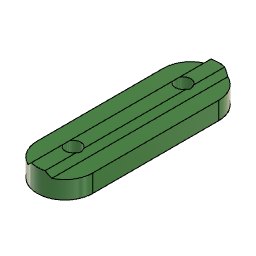
v2020_z_6_4mmshim_plate_v3 (Autodesk Fusion 360 design; units mm, degrees)
Autodesk Fusion 360 part; units mm, degrees
sketch "Sketch1" plane through (0, 0, 0) normal (0, 0, 1) x (1, 0, 0)
  circle A0 centre (0, -19.85) radius 2.8
  circle A1 centre (0, -10) radius 2.55 construction
  circle A2 centre (0, 0) radius 2.55 construction
  circle A3 centre (0, 10) radius 2.55 construction
  circle A4 centre (0, 19.85) radius 2.8
  circle A5 centre (-10, 0) radius 2.55 construction
  circle A6 centre (-10, 19.85) radius 2.55 construction
  circle A7 centre (-10, -19.85) radius 2.55 construction
  circle A8 centre (10, -19.85) radius 2.55 construction
  circle A9 centre (10, 0) radius 2.55 construction
  circle A10 centre (10, 19.85) radius 2.55 construction
  circle A11 centre (-20, -19.85) radius 3.6
  circle A12 centre (-20, 19.85) radius 2.55
  circle A13 centre (20, 19.85) radius 2.55
  circle A14 centre (20, -19.85) radius 3.6
  line L0 (-32.75, 29.75) -> (-32.75, -29.75)
  arc A15 (-32.75, -29.75) -> (-29.75, -32.75) centre (-29.75, -29.75) ccw
  line L1 (0, -32.75) -> (0, -32.75)
  arc A16 (-29.75, 32.75) -> (-32.75, 29.75) centre (-29.75, 29.75) ccw
  line L2 (0, 32.75) -> (0, 32.75)
  arc A17 (32.75, 29.75) -> (29.75, 32.75) centre (29.75, 29.75) ccw
  line L3 (32.75, -29.75) -> (32.75, 29.75)
  arc A18 (29.75, -32.75) -> (32.75, -29.75) centre (29.75, -29.75) ccw
  line L4 (26.2, -23.4) -> (26.2, -16.9)
  line L5 (29.2, -16.9) -> (29.2, -23.4)
  line L6 (29.2, 3.25) -> (29.2, -3.25)
  line L7 (26.2, -3.25) -> (26.2, 3.25)
  line L8 (26.2, 16.9) -> (26.2, 23.4)
  line L9 (29.2, 23.4) -> (29.2, 16.9)
  arc A19 (29.2, 23.4) -> (26.2, 23.4) centre (27.7, 23.4) ccw
  arc A20 (26.2, 16.9) -> (29.2, 16.9) centre (27.7, 16.9) ccw
  arc A21 (29.2, 3.25) -> (26.2, 3.25) centre (27.7, 3.25) ccw
  arc A22 (26.2, -3.25) -> (29.2, -3.25) centre (27.7, -3.25) ccw
  arc A23 (29.2, -16.9) -> (26.2, -16.9) centre (27.7, -16.9) ccw
  arc A24 (26.2, -23.4) -> (29.2, -23.4) centre (27.7, -23.4) ccw
  arc A25 (17.5, -10.32) -> (22.5, -10.32) centre (20, -10.32) ccw
  arc A26 (22.5, 10.32) -> (17.5, 10.32) centre (20, 10.32) ccw
  line L10 (17.5, -10.32) -> (17.5, 10.32)
  line L11 (22.5, 10.32) -> (22.5, -10.32)
  arc A27 (-17.5, 10.32) -> (-22.5, 10.32) centre (-20, 10.32) ccw
  arc A28 (-22.5, -10.32) -> (-17.5, -10.32) centre (-20, -10.32) ccw
  line L12 (-17.5, 10.32) -> (-17.5, -10.32)
  line L13 (-22.5, -10.32) -> (-22.5, 10.32)
  arc A29 (-26.2, 3.25) -> (-29.2, 3.25) centre (-27.7, 3.25) ccw
  arc A30 (-29.2, -3.25) -> (-26.2, -3.25) centre (-27.7, -3.25) ccw
  line L14 (-29.2, -3.25) -> (-29.2, 3.25)
  line L15 (-26.2, 3.25) -> (-26.2, -3.25)
  arc A31 (-26.2, -16.9) -> (-29.2, -16.9) centre (-27.7, -16.9) ccw
  arc A32 (-29.2, -23.4) -> (-26.2, -23.4) centre (-27.7, -23.4) ccw
  line L16 (-26.2, -16.9) -> (-26.2, -23.4)
  line L17 (-29.2, -23.4) -> (-29.2, -16.9)
  arc A33 (-29.2, 16.9) -> (-26.2, 16.9) centre (-27.7, 16.9) ccw
  arc A34 (-26.2, 23.4) -> (-29.2, 23.4) centre (-27.7, 23.4) ccw
  line L18 (-29.2, 16.9) -> (-29.2, 23.4)
  line L19 (-26.2, 23.4) -> (-26.2, 16.9)
  line L20 (0, 32.75) -> (0, -32.75) construction
  line L21 (-10, 32.75) -> (-10, -32.75)
  line L22 (10, 32.75) -> (10, -32.75)
  arc A35 (-9.9939, -22.4) -> (9.9939, -22.4) centre (0, -22.75) ccw
  arc A36 (9.9939, 22.4) -> (-9.9939, 22.4) centre (0, 22.75) ccw
  line L23 (-29.75, -32.75) -> (29.75, -32.75)
  line L24 (-29.75, 32.75) -> (29.75, 32.75)
  dimension "d3" = 5.6
  dimension "d4" = 5.6
  constraint parallel L20 L21
  constraint parallel L20 L22
  constraint coincident A18.start L1
  constraint coincident A17.end L2
  constraint tangent L22 A36
  constraint coincident A7 A35.start
  constraint coincident A8 A35.end
  constraint coincident A6 A36.end
  constraint coincident A10 A36.start
  constraint tangent A18 L23
  constraint tangent A17 L24
  measures "d3" diameter of A4
  measures "d4" diameter of A0 A14.centre
sketch "Sketch2" plane through (0, 0, 0) normal (0, 1, 0) x (1, 0, 0)
  line L0 (4.2864, -6.4) -> (-4.2864, -6.4)
  line L1 (4.2864, -6.4) -> (2.4864, -8.2)
  line L2 (2.4864, -24.6) -> (-2.4864, -24.6)
  line L3 (-2.4864, -8.2) -> (-4.2864, -6.4)
  circle A0 centre (0, -16.4) radius 2.1 construction
  line L4 (2.4864, -8.2) -> (-2.4864, -8.2)
  line L5 (4.2864, -26.4) -> (2.4864, -24.6)
  line L6 (4.2864, -26.4) -> (-4.2864, -26.4)
  line L7 (-2.4864, -24.6) -> (-4.2864, -26.4)
  line L8 (3.9, -19.24) -> (3.9, -13.56) construction
  line L9 (-6.56, -21.9) -> (-8.2, -21.9) construction
  line L10 (8.2, -19.24) -> (8.2, -21.9) construction
  line L11 (-3.9, -13.56) -> (-3.9, -19.24) construction
  line L12 (8.2, -21.9) -> (6.56, -21.9) construction
  line L13 (-5.5, -24.6) -> (-5.5, -22.96) construction
  line L14 (2.84, -12.5) -> (-2.84, -12.5) construction
  line L15 (10, -26.4) -> (10, -21.04) construction
  line L16 (6.56, -10.9) -> (8.2, -10.9) construction
  line L17 (6.56, -21.9) -> (3.9, -19.24) construction
  line L18 (5.5, -24.6) -> (2.84, -24.6) construction
  line L19 (-2.84, -12.5) -> (-5.5, -9.84) construction
  line L20 (-2.84, -24.6) -> (-5.5, -24.6) construction
  line L21 (-3.9, -19.24) -> (-6.56, -21.9) construction
  line L22 (-6.56, -10.9) -> (-3.9, -13.56) construction
  line L23 (-5.5, -22.96) -> (-2.84, -20.3) construction
  line L24 (-10, -26.4) -> (-4.64, -26.4) construction
  line L25 (-5.5, -8.2) -> (-2.84, -8.2) construction
  line L26 (-4.64, -6.4) -> (-10, -6.4) construction
  line L27 (-8.2, -13.56) -> (-8.2, -10.9) construction
  line L28 (5.5, -9.84) -> (2.84, -12.5) construction
  line L29 (-8.2, -10.9) -> (-6.56, -10.9) construction
  line L30 (-10, -6.4) -> (-10, -11.76) construction
  line L31 (5.5, -8.2) -> (5.5, -9.84) construction
  line L32 (-10, -11.76) -> (-8.2, -13.56) construction
  line L33 (10, -21.04) -> (8.2, -19.24) construction
  line L34 (-2.84, -20.3) -> (2.84, -20.3) construction
  line L35 (-8.2, -19.24) -> (-10, -21.04) construction
  line L36 (-8.2, -21.9) -> (-8.2, -19.24) construction
  line L37 (2.84, -8.2) -> (5.5, -8.2) construction
  line L38 (-10, -21.04) -> (-10, -26.4) construction
  line L39 (8.2, -10.9) -> (8.2, -13.56) construction
  line L40 (2.84, -24.6) -> (4.64, -26.4) construction
  line L41 (-5.5, -9.84) -> (-5.5, -8.2) construction
  line L42 (3.9, -13.56) -> (6.56, -10.9) construction
  line L43 (4.64, -26.4) -> (10, -26.4) construction
  line L44 (10, -6.4) -> (4.64, -6.4) construction
  line L45 (5.5, -22.96) -> (5.5, -24.6) construction
  line L46 (2.84, -20.3) -> (5.5, -22.96) construction
  line L47 (-4.64, -26.4) -> (-2.84, -24.6) construction
  line L48 (10, -11.76) -> (10, -6.4) construction
  line L49 (-2.84, -8.2) -> (-4.64, -6.4) construction
  line L50 (8.2, -13.56) -> (10, -11.76) construction
  line L51 (4.64, -6.4) -> (2.84, -8.2) construction
extrude "Extrude1" add sketch "Sketch1" along normal blind 6.4 contours L21 L22 A35 A36
extrude "Extrude2" add sketch "Sketch2" along normal mid plane 65.5 contours L0 L1 L3 L4
extrude "Extrude3" cut sketch "Sketch1" along normal through all contours A0 | A4
extrude "Extrude4" cut sketch "Sketch1" along normal through all contours L21 A36 L24 | L21 A35 L23 | L22 A36 L24 | L22 A35 L23
named bodies: "V2020_Z_6_4mmShim_Plate"
